Autodesk Fusion 360 part; units mm, degrees
(part 6 of 14)
  line L3010 (-202.4856, -153.9875) -> (-196.9863, -163.5125)
  line L3011 (-196.9863, -163.5125) -> (-185.9878, -163.5125)
  line L3012 (-180.4886, -153.9875) -> (-185.9878, -144.4625)
  line L3013 (-185.9878, -163.5125) -> (-180.4886, -153.9875)
  line L3014 (-166.7404, -133.35) -> (-177.7389, -133.35)
  line L3015 (-177.7389, -133.35) -> (-183.2382, -142.875)
  line L3016 (-183.2382, -142.875) -> (-177.7389, -152.4)
  line L3017 (-177.7389, -152.4) -> (-166.7404, -152.4)
  line L3018 (-161.2411, -142.875) -> (-166.7404, -133.35)
  line L3019 (-166.7404, -152.4) -> (-161.2411, -142.875)
  line L3020 (-147.493, -122.2375) -> (-158.4915, -122.2375)
  line L3021 (-158.4915, -122.2375) -> (-163.9908, -131.7625)
  line L3022 (-163.9908, -131.7625) -> (-158.4915, -141.2875)
  line L3023 (-158.4915, -141.2875) -> (-147.493, -141.2875)
  line L3024 (-141.9937, -131.7625) -> (-147.493, -122.2375)
  line L3025 (-147.493, -141.2875) -> (-141.9937, -131.7625)
  line L3026 (-128.2456, -111.125) -> (-139.2441, -111.125)
  line L3027 (-139.2441, -111.125) -> (-144.7434, -120.65)
  line L3028 (-144.7434, -120.65) -> (-139.2441, -130.175)
  line L3029 (-139.2441, -130.175) -> (-128.2456, -130.175)
  line L3030 (-122.7463, -120.65) -> (-128.2456, -111.125)
  line L3031 (-128.2456, -130.175) -> (-122.7463, -120.65)
  line L3032 (-108.9982, -100.0125) -> (-119.9967, -100.0125)
  line L3033 (-119.9967, -100.0125) -> (-125.4959, -109.5375)
  line L3034 (-125.4959, -109.5375) -> (-119.9967, -119.0625)
  line L3035 (-119.9967, -119.0625) -> (-108.9982, -119.0625)
  line L3036 (-103.4989, -109.5375) -> (-108.9982, -100.0125)
  line L3037 (-108.9982, -119.0625) -> (-103.4989, -109.5375)
  line L3038 (-89.7507, -88.9) -> (-100.7493, -88.9)
  line L3039 (-100.7493, -88.9) -> (-106.2485, -98.425)
  line L3040 (-106.2485, -98.425) -> (-100.7493, -107.95)
  line L3041 (-100.7493, -107.95) -> (-89.7507, -107.95)
  line L3042 (-84.2515, -98.425) -> (-89.7507, -88.9)
  line L3043 (-89.7507, -107.95) -> (-84.2515, -98.425)
  line L3044 (-70.5033, -77.7875) -> (-81.5018, -77.7875)
  line L3045 (-81.5018, -77.7875) -> (-87.0011, -87.3125)
  line L3046 (-87.0011, -87.3125) -> (-81.5018, -96.8375)
  line L3047 (-81.5018, -96.8375) -> (-70.5033, -96.8375)
  line L3048 (-65.0041, -87.3125) -> (-70.5033, -77.7875)
  line L3049 (-70.5033, -96.8375) -> (-65.0041, -87.3125)
  line L3050 (-51.2559, -66.675) -> (-62.2544, -66.675)
  line L3051 (-62.2544, -66.675) -> (-67.7537, -76.2)
  line L3052 (-67.7537, -76.2) -> (-62.2544, -85.725)
  line L3053 (-62.2544, -85.725) -> (-51.2559, -85.725)
  line L3054 (-45.7566, -76.2) -> (-51.2559, -66.675)
  line L3055 (-51.2559, -85.725) -> (-45.7566, -76.2)
  line L3056 (-32.0085, -55.5625) -> (-43.007, -55.5625)
  line L3057 (-43.007, -55.5625) -> (-48.5063, -65.0875)
  line L3058 (-48.5063, -65.0875) -> (-43.007, -74.6125)
  line L3059 (-43.007, -74.6125) -> (-32.0085, -74.6125)
  line L3060 (-26.5092, -65.0875) -> (-32.0085, -55.5625)
  line L3061 (-32.0085, -74.6125) -> (-26.5092, -65.0875)
  line L3062 (-12.7611, -44.45) -> (-23.7596, -44.45)
  line L3063 (-23.7596, -44.45) -> (-29.2589, -53.975)
  line L3064 (-29.2589, -53.975) -> (-23.7596, -63.5)
  line L3065 (-23.7596, -63.5) -> (-12.7611, -63.5)
  line L3066 (-7.2618, -53.975) -> (-12.7611, -44.45)
  line L3067 (-12.7611, -63.5) -> (-7.2618, -53.975)
  line L3068 (6.4863, -33.3375) -> (-4.5122, -33.3375)
  line L3069 (-4.5122, -33.3375) -> (-10.0114, -42.8625)
  line L3070 (-10.0114, -42.8625) -> (-4.5122, -52.3875)
  line L3071 (-4.5122, -52.3875) -> (6.4863, -52.3875)
  line L3072 (11.9856, -42.8625) -> (6.4863, -33.3375)
  line L3073 (6.4863, -52.3875) -> (11.9856, -42.8625)
  line L3074 (25.7337, -22.225) -> (14.7352, -22.225)
  line L3075 (14.7352, -22.225) -> (9.236, -31.75)
  line L3076 (9.236, -31.75) -> (14.7352, -41.275)
  line L3077 (14.7352, -41.275) -> (25.7337, -41.275)
  line L3078 (31.233, -31.75) -> (25.7337, -22.225)
  line L3079 (25.7337, -41.275) -> (31.233, -31.75)
  line L3080 (44.9812, -11.1125) -> (33.9826, -11.1125)
  line L3081 (33.9826, -11.1125) -> (28.4834, -20.6375)
  line L3082 (28.4834, -20.6375) -> (33.9826, -30.1625)
  line L3083 (33.9826, -30.1625) -> (44.9812, -30.1625)
  line L3084 (50.4804, -20.6375) -> (44.9812, -11.1125)
  line L3085 (44.9812, -30.1625) -> (50.4804, -20.6375)
  line L3086 (64.2286, 0) -> (53.2301, 0)
  line L3087 (53.2301, 0) -> (47.7308, -9.525)
  line L3088 (47.7308, -9.525) -> (53.2301, -19.05)
  line L3089 (53.2301, -19.05) -> (64.2286, -19.05)
  line L3090 (69.7278, -9.525) -> (64.2286, 0)
  line L3091 (64.2286, -19.05) -> (69.7278, -9.525)
  line L3092 (83.476, 11.1125) -> (72.4775, 11.1125)
  line L3093 (72.4775, 11.1125) -> (66.9782, 1.5875)
  line L3094 (66.9782, 1.5875) -> (72.4775, -7.9375)
  line L3095 (72.4775, -7.9375) -> (83.476, -7.9375)
  line L3096 (88.9753, 1.5875) -> (83.476, 11.1125)
  line L3097 (83.476, -7.9375) -> (88.9753, 1.5875)
  line L3098 (102.7234, 22.225) -> (91.7249, 22.225)
  line L3099 (91.7249, 22.225) -> (86.2256, 12.7)
  line L3100 (86.2256, 12.7) -> (91.7249, 3.175)
  line L3101 (91.7249, 3.175) -> (102.7234, 3.175)
  line L3102 (108.2227, 12.7) -> (102.7234, 22.225)
  line L3103 (102.7234, 3.175) -> (108.2227, 12.7)
  line L3104 (121.9708, 33.3375) -> (110.9723, 33.3375)
  line L3105 (110.9723, 33.3375) -> (105.473, 23.8125)
  line L3106 (105.473, 23.8125) -> (110.9723, 14.2875)
  line L3107 (110.9723, 14.2875) -> (121.9708, 14.2875)
  line L3108 (127.4701, 23.8125) -> (121.9708, 33.3375)
  line L3109 (121.9708, 14.2875) -> (127.4701, 23.8125)
  line L3110 (141.2182, 44.45) -> (130.2197, 44.45)
  line L3111 (130.2197, 44.45) -> (124.7205, 34.925)
  line L3112 (124.7205, 34.925) -> (130.2197, 25.4)
  line L3113 (130.2197, 25.4) -> (141.2182, 25.4)
  line L3114 (146.7175, 34.925) -> (141.2182, 44.45)
  line L3115 (141.2182, 25.4) -> (146.7175, 34.925)
  line L3116 (160.4657, 55.5625) -> (149.4671, 55.5625)
  line L3117 (149.4671, 55.5625) -> (143.9679, 46.0375)
  line L3118 (143.9679, 46.0375) -> (149.4671, 36.5125)
  line L3119 (149.4671, 36.5125) -> (160.4657, 36.5125)
  line L3120 (165.9649, 46.0375) -> (160.4657, 55.5625)
  line L3121 (160.4657, 36.5125) -> (165.9649, 46.0375)
  line L3122 (179.7131, 66.675) -> (168.7145, 66.675)
  line L3123 (168.7145, 66.675) -> (163.2153, 57.15)
  line L3124 (163.2153, 57.15) -> (168.7145, 47.625)
  line L3125 (168.7145, 47.625) -> (179.7131, 47.625)
  line L3126 (185.2123, 57.15) -> (179.7131, 66.675)
  line L3127 (179.7131, 47.625) -> (185.2123, 57.15)
  line L3128 (198.9605, 77.7875) -> (187.962, 77.7875)
  line L3129 (187.962, 77.7875) -> (182.4627, 68.2625)
  line L3130 (182.4627, 68.2625) -> (187.962, 58.7375)
  line L3131 (187.962, 58.7375) -> (198.9605, 58.7375)
  line L3132 (204.4597, 68.2625) -> (198.9605, 77.7875)
  line L3133 (198.9605, 58.7375) -> (204.4597, 68.2625)
  line L3134 (218.2079, 88.9) -> (207.2094, 88.9)
  line L3135 (207.2094, 88.9) -> (201.7101, 79.375)
  line L3136 (201.7101, 79.375) -> (207.2094, 69.85)
  line L3137 (207.2094, 69.85) -> (218.2079, 69.85)
  line L3138 (223.7072, 79.375) -> (218.2079, 88.9)
  line L3139 (218.2079, 69.85) -> (223.7072, 79.375)
  line L3140 (237.4553, 100.0125) -> (226.4568, 100.0125)
  line L3141 (226.4568, 100.0125) -> (220.9575, 90.4875)
  line L3142 (220.9575, 90.4875) -> (226.4568, 80.9625)
  line L3143 (226.4568, 80.9625) -> (237.4553, 80.9625)
  line L3144 (242.9546, 90.4875) -> (237.4553, 100.0125)
  line L3145 (237.4553, 80.9625) -> (242.9546, 90.4875)
  line L3146 (256.7027, 111.125) -> (245.7042, 111.125)
  line L3147 (245.7042, 111.125) -> (240.2049, 101.6)
  line L3148 (240.2049, 101.6) -> (245.7042, 92.075)
  line L3149 (245.7042, 92.075) -> (256.7027, 92.075)
  line L3150 (262.202, 101.6) -> (256.7027, 111.125)
  line L3151 (256.7027, 92.075) -> (262.202, 101.6)
  line L3152 (275.9501, 122.2375) -> (264.9516, 122.2375)
  line L3153 (264.9516, 122.2375) -> (259.4524, 112.7125)
  line L3154 (259.4524, 112.7125) -> (264.9516, 103.1875)
  line L3155 (264.9516, 103.1875) -> (275.9501, 103.1875)
  line L3156 (281.4494, 112.7125) -> (275.9501, 122.2375)
  line L3157 (275.9501, 103.1875) -> (281.4494, 112.7125)
  line L3158 (295.1976, 133.35) -> (284.199, 133.35)
  line L3159 (284.199, 133.35) -> (278.6998, 123.825)
  line L3160 (278.6998, 123.825) -> (284.199, 114.3)
  line L3161 (284.199, 114.3) -> (295.1976, 114.3)
  line L3162 (300.6968, 123.825) -> (295.1976, 133.35)
  line L3163 (295.1976, 114.3) -> (300.6968, 123.825)
  line L3164 (314.445, 144.4625) -> (303.4464, 144.4625)
  line L3165 (303.4464, 144.4625) -> (297.9472, 134.9375)
  line L3166 (297.9472, 134.9375) -> (303.4464, 125.4125)
  line L3167 (303.4464, 125.4125) -> (314.445, 125.4125)
  line L3168 (319.9442, 134.9375) -> (314.445, 144.4625)
  line L3169 (314.445, 125.4125) -> (319.9442, 134.9375)
  line L3170 (333.6924, 155.575) -> (322.6939, 155.575)
  line L3171 (322.6939, 155.575) -> (317.1946, 146.05)
  line L3172 (317.1946, 146.05) -> (322.6939, 136.525)
  line L3173 (322.6939, 136.525) -> (333.6924, 136.525)
  line L3174 (339.1916, 146.05) -> (333.6924, 155.575)
  line L3175 (333.6924, 136.525) -> (339.1916, 146.05)
  line L3176 (352.9398, 166.6875) -> (341.9413, 166.6875)
  line L3177 (341.9413, 166.6875) -> (336.442, 157.1625)
  line L3178 (336.442, 157.1625) -> (341.9413, 147.6375)
  line L3179 (341.9413, 147.6375) -> (352.9398, 147.6375)
  line L3180 (358.4391, 157.1625) -> (352.9398, 166.6875)
  line L3181 (352.9398, 147.6375) -> (358.4391, 157.1625)
  line L3182 (372.1872, 177.8) -> (361.1887, 177.8)
  line L3183 (361.1887, 177.8) -> (355.6894, 168.275)
  line L3184 (355.6894, 168.275) -> (361.1887, 158.75)
  line L3185 (361.1887, 158.75) -> (372.1872, 158.75)
  line L3186 (377.6865, 168.275) -> (372.1872, 177.8)
  line L3187 (372.1872, 158.75) -> (377.6865, 168.275)
  line L3188 (391.4346, 188.9125) -> (380.4361, 188.9125)
  line L3189 (380.4361, 188.9125) -> (374.9368, 179.3875)
  line L3190 (374.9368, 179.3875) -> (380.4361, 169.8625)
  line L3191 (380.4361, 169.8625) -> (391.4346, 169.8625)
  line L3192 (396.9339, 179.3875) -> (391.4346, 188.9125)
  line L3193 (391.4346, 169.8625) -> (396.9339, 179.3875)
  line L3194 (410.682, 200.025) -> (399.6835, 200.025)
  line L3195 (399.6835, 200.025) -> (394.1843, 190.5)
  line L3196 (394.1843, 190.5) -> (399.6835, 180.975)
  line L3197 (399.6835, 180.975) -> (410.682, 180.975)
  line L3198 (416.1813, 190.5) -> (410.682, 200.025)
  line L3199 (410.682, 180.975) -> (416.1813, 190.5)
  line L3200 (429.9295, 211.1375) -> (418.9309, 211.1375)
  line L3201 (418.9309, 211.1375) -> (413.4317, 201.6125)
  line L3202 (413.4317, 201.6125) -> (418.9309, 192.0875)
  line L3203 (418.9309, 192.0875) -> (429.9295, 192.0875)
  line L3204 (435.4287, 201.6125) -> (429.9295, 211.1375)
  line L3205 (429.9295, 192.0875) -> (435.4287, 201.6125)
  line L3206 (449.1769, 222.25) -> (438.1783, 222.25)
  line L3207 (438.1783, 222.25) -> (432.6791, 212.725)
  line L3208 (432.6791, 212.725) -> (438.1783, 203.2)
  line L3209 (438.1783, 203.2) -> (449.1769, 203.2)
  line L3210 (454.6761, 212.725) -> (449.1769, 222.25)
  line L3211 (449.1769, 203.2) -> (454.6761, 212.725)
  line L3212 (468.4243, 233.3625) -> (457.4258, 233.3625)
  line L3213 (457.4258, 233.3625) -> (451.9265, 223.8375)
  line L3214 (451.9265, 223.8375) -> (457.4258, 214.3125)
  line L3215 (457.4258, 214.3125) -> (468.4243, 214.3125)
  line L3216 (473.9235, 223.8375) -> (468.4243, 233.3625)
  line L3217 (468.4243, 214.3125) -> (473.9235, 223.8375)
  line L3218 (487.6717, 244.475) -> (476.6732, 244.475)
  line L3219 (476.6732, 244.475) -> (471.1739, 234.95)
  line L3220 (471.1739, 234.95) -> (476.6732, 225.425)
  line L3221 (476.6732, 225.425) -> (487.6717, 225.425)
  line L3222 (493.171, 234.95) -> (487.6717, 244.475)
  line L3223 (487.6717, 225.425) -> (493.171, 234.95)
  line L3224 (506.9191, 255.5875) -> (495.9206, 255.5875)
  line L3225 (495.9206, 255.5875) -> (490.4213, 246.0625)
  line L3226 (490.4213, 246.0625) -> (495.9206, 236.5375)
  line L3227 (495.9206, 236.5375) -> (506.9191, 236.5375)
  line L3228 (512.4184, 246.0625) -> (506.9191, 255.5875)
  line L3229 (506.9191, 236.5375) -> (512.4184, 246.0625)
  line L3230 (526.1665, 266.7) -> (515.168, 266.7)
  line L3231 (515.168, 266.7) -> (509.6687, 257.175)
  line L3232 (509.6687, 257.175) -> (515.168, 247.65)
  line L3233 (515.168, 247.65) -> (526.1665, 247.65)
  line L3234 (531.6658, 257.175) -> (526.1665, 266.7)
  line L3235 (526.1665, 247.65) -> (531.6658, 257.175)
  line L3236 (545.4139, 277.8125) -> (534.4154, 277.8125)
  line L3237 (534.4154, 277.8125) -> (528.9162, 268.2875)
  line L3238 (528.9162, 268.2875) -> (534.4154, 258.7625)
  line L3239 (534.4154, 258.7625) -> (545.4139, 258.7625)
  line L3240 (550.9132, 268.2875) -> (545.4139, 277.8125)
  line L3241 (545.4139, 258.7625) -> (550.9132, 268.2875)
  line L3242 (564.6614, 288.925) -> (553.6628, 288.925)
  line L3243 (553.6628, 288.925) -> (548.1636, 279.4)
  line L3244 (548.1636, 279.4) -> (553.6628, 269.875)
  line L3245 (553.6628, 269.875) -> (564.6614, 269.875)
  line L3246 (570.1606, 279.4) -> (564.6614, 288.925)
  line L3247 (564.6614, 269.875) -> (570.1606, 279.4)
  line L3248 (583.9088, 300.0375) -> (572.9102, 300.0375)
  line L3249 (572.9102, 300.0375) -> (567.411, 290.5125)
  line L3250 (567.411, 290.5125) -> (572.9102, 280.9875)
  line L3251 (572.9102, 280.9875) -> (583.9088, 280.9875)
  line L3252 (589.408, 290.5125) -> (583.9088, 300.0375)
  line L3253 (583.9088, 280.9875) -> (589.408, 290.5125)
  line L3254 (603.1562, 311.15) -> (592.1577, 311.15)
  line L3255 (592.1577, 311.15) -> (586.6584, 301.625)
  line L3256 (586.6584, 301.625) -> (592.1577, 292.1)
  line L3257 (592.1577, 292.1) -> (603.1562, 292.1)
  line L3258 (608.6554, 301.625) -> (603.1562, 311.15)
  line L3259 (603.1562, 292.1) -> (608.6554, 301.625)
  line L3260 (-551.6887, -333.375) -> (-562.6872, -333.375)
  line L3261 (-562.6872, -333.375) -> (-568.1865, -342.9)
  line L3262 (-568.1865, -342.9) -> (-562.6872, -352.425)
  line L3263 (-562.6872, -352.425) -> (-551.6887, -352.425)
  line L3264 (-546.1894, -342.9) -> (-551.6887, -333.375)
  line L3265 (-551.6887, -352.425) -> (-546.1894, -342.9)
  line L3266 (-532.4413, -322.2625) -> (-543.4398, -322.2625)
  line L3267 (-543.4398, -322.2625) -> (-548.9391, -331.7875)
  line L3268 (-548.9391, -331.7875) -> (-543.4398, -341.3125)
  line L3269 (-543.4398, -341.3125) -> (-532.4413, -341.3125)
  line L3270 (-526.942, -331.7875) -> (-532.4413, -322.2625)
  line L3271 (-532.4413, -341.3125) -> (-526.942, -331.7875)
  line L3272 (-513.1939, -311.15) -> (-524.1924, -311.15)
  line L3273 (-524.1924, -311.15) -> (-529.6916, -320.675)
  line L3274 (-529.6916, -320.675) -> (-524.1924, -330.2)
  line L3275 (-524.1924, -330.2) -> (-513.1939, -330.2)
  line L3276 (-507.6946, -320.675) -> (-513.1939, -311.15)
  line L3277 (-513.1939, -330.2) -> (-507.6946, -320.675)
  line L3278 (-493.9464, -300.0375) -> (-504.945, -300.0375)
  line L3279 (-504.945, -300.0375) -> (-510.4442, -309.5625)
  line L3280 (-510.4442, -309.5625) -> (-504.945, -319.0875)
  line L3281 (-504.945, -319.0875) -> (-493.9464, -319.0875)
  line L3282 (-488.4472, -309.5625) -> (-493.9464, -300.0375)
  line L3283 (-493.9464, -319.0875) -> (-488.4472, -309.5625)
  line L3284 (-474.699, -288.925) -> (-485.6976, -288.925)
  line L3285 (-485.6976, -288.925) -> (-491.1968, -298.45)
  line L3286 (-491.1968, -298.45) -> (-485.6976, -307.975)
  line L3287 (-485.6976, -307.975) -> (-474.699, -307.975)
  line L3288 (-469.1998, -298.45) -> (-474.699, -288.925)
  line L3289 (-474.699, -307.975) -> (-469.1998, -298.45)
  line L3290 (-455.4516, -277.8125) -> (-466.4501, -277.8125)
  line L3291 (-466.4501, -277.8125) -> (-471.9494, -287.3375)
  line L3292 (-471.9494, -287.3375) -> (-466.4501, -296.8625)
  line L3293 (-466.4501, -296.8625) -> (-455.4516, -296.8625)
  line L3294 (-449.9524, -287.3375) -> (-455.4516, -277.8125)
  line L3295 (-455.4516, -296.8625) -> (-449.9524, -287.3375)
  line L3296 (-436.2042, -266.7) -> (-447.2027, -266.7)
  line L3297 (-447.2027, -266.7) -> (-452.702, -276.225)
  line L3298 (-452.702, -276.225) -> (-447.2027, -285.75)
  line L3299 (-447.2027, -285.75) -> (-436.2042, -285.75)
  line L3300 (-430.7049, -276.225) -> (-436.2042, -266.7)
  line L3301 (-436.2042, -285.75) -> (-430.7049, -276.225)
  line L3302 (-416.9568, -255.5875) -> (-427.9553, -255.5875)
  line L3303 (-427.9553, -255.5875) -> (-433.4546, -265.1125)
  line L3304 (-433.4546, -265.1125) -> (-427.9553, -274.6375)
  line L3305 (-427.9553, -274.6375) -> (-416.9568, -274.6375)
  line L3306 (-411.4575, -265.1125) -> (-416.9568, -255.5875)
  line L3307 (-416.9568, -274.6375) -> (-411.4575, -265.1125)
  line L3308 (-397.7094, -244.475) -> (-408.7079, -244.475)
  line L3309 (-408.7079, -244.475) -> (-414.2072, -254)
  line L3310 (-414.2072, -254) -> (-408.7079, -263.525)
  line L3311 (-408.7079, -263.525) -> (-397.7094, -263.525)
  line L3312 (-392.2101, -254) -> (-397.7094, -244.475)
  line L3313 (-397.7094, -263.525) -> (-392.2101, -254)
  line L3314 (-378.462, -233.3625) -> (-389.4605, -233.3625)
  line L3315 (-389.4605, -233.3625) -> (-394.9597, -242.8875)
  line L3316 (-394.9597, -242.8875) -> (-389.4605, -252.4125)
  line L3317 (-389.4605, -252.4125) -> (-378.462, -252.4125)
  line L3318 (-372.9627, -242.8875) -> (-378.462, -233.3625)
  line L3319 (-378.462, -252.4125) -> (-372.9627, -242.8875)
  line L3320 (-359.2145, -222.25) -> (-370.2131, -222.25)
  line L3321 (-370.2131, -222.25) -> (-375.7123, -231.775)
  line L3322 (-375.7123, -231.775) -> (-370.2131, -241.3)
  line L3323 (-370.2131, -241.3) -> (-359.2145, -241.3)
  line L3324 (-353.7153, -231.775) -> (-359.2145, -222.25)
  line L3325 (-359.2145, -241.3) -> (-353.7153, -231.775)
  line L3326 (-339.9671, -211.1375) -> (-350.9657, -211.1375)
  line L3327 (-350.9657, -211.1375) -> (-356.4649, -220.6625)
  line L3328 (-356.4649, -220.6625) -> (-350.9657, -230.1875)
  line L3329 (-350.9657, -230.1875) -> (-339.9671, -230.1875)
  line L3330 (-334.4679, -220.6625) -> (-339.9671, -211.1375)
  line L3331 (-339.9671, -230.1875) -> (-334.4679, -220.6625)
  line L3332 (-320.7197, -200.025) -> (-331.7182, -200.025)
  line L3333 (-331.7182, -200.025) -> (-337.2175, -209.55)
  line L3334 (-337.2175, -209.55) -> (-331.7182, -219.075)
  line L3335 (-331.7182, -219.075) -> (-320.7197, -219.075)
  line L3336 (-315.2205, -209.55) -> (-320.7197, -200.025)
  line L3337 (-320.7197, -219.075) -> (-315.2205, -209.55)
  line L3338 (-301.4723, -188.9125) -> (-312.4708, -188.9125)
  line L3339 (-312.4708, -188.9125) -> (-317.9701, -198.4375)
  line L3340 (-317.9701, -198.4375) -> (-312.4708, -207.9625)
  line L3341 (-312.4708, -207.9625) -> (-301.4723, -207.9625)
  line L3342 (-295.973, -198.4375) -> (-301.4723, -188.9125)
  line L3343 (-301.4723, -207.9625) -> (-295.973, -198.4375)
  line L3344 (-282.2249, -177.8) -> (-293.2234, -177.8)
  line L3345 (-293.2234, -177.8) -> (-298.7227, -187.325)
  line L3346 (-298.7227, -187.325) -> (-293.2234, -196.85)
  line L3347 (-293.2234, -196.85) -> (-282.2249, -196.85)
  line L3348 (-276.7256, -187.325) -> (-282.2249, -177.8)
  line L3349 (-282.2249, -196.85) -> (-276.7256, -187.325)
  line L3350 (-262.9775, -166.6875) -> (-273.976, -166.6875)
  line L3351 (-273.976, -166.6875) -> (-279.4753, -176.2125)
  line L3352 (-279.4753, -176.2125) -> (-273.976, -185.7375)
  line L3353 (-273.976, -185.7375) -> (-262.9775, -185.7375)
  line L3354 (-257.4782, -176.2125) -> (-262.9775, -166.6875)
  line L3355 (-262.9775, -185.7375) -> (-257.4782, -176.2125)
  line L3356 (-243.7301, -155.575) -> (-254.7286, -155.575)
  line L3357 (-254.7286, -155.575) -> (-260.2278, -165.1)
  line L3358 (-260.2278, -165.1) -> (-254.7286, -174.625)
  line L3359 (-254.7286, -174.625) -> (-243.7301, -174.625)
  line L3360 (-238.2308, -165.1) -> (-243.7301, -155.575)
  line L3361 (-243.7301, -174.625) -> (-238.2308, -165.1)
  line L3362 (-224.4826, -144.4625) -> (-235.4812, -144.4625)
  line L3363 (-235.4812, -144.4625) -> (-240.9804, -153.9875)
  line L3364 (-240.9804, -153.9875) -> (-235.4812, -163.5125)
  line L3365 (-235.4812, -163.5125) -> (-224.4826, -163.5125)
  line L3366 (-218.9834, -153.9875) -> (-224.4826, -144.4625)
  line L3367 (-224.4826, -163.5125) -> (-218.9834, -153.9875)
  line L3368 (-205.2352, -133.35) -> (-216.2337, -133.35)
  line L3369 (-216.2337, -133.35) -> (-221.733, -142.875)
  line L3370 (-221.733, -142.875) -> (-216.2337, -152.4)
  line L3371 (-216.2337, -152.4) -> (-205.2352, -152.4)
  line L3372 (-199.736, -142.875) -> (-205.2352, -133.35)
  line L3373 (-205.2352, -152.4) -> (-199.736, -142.875)
  line L3374 (-185.9878, -122.2375) -> (-196.9863, -122.2375)
  line L3375 (-196.9863, -122.2375) -> (-202.4856, -131.7625)
  line L3376 (-202.4856, -131.7625) -> (-196.9863, -141.2875)
  line L3377 (-196.9863, -141.2875) -> (-185.9878, -141.2875)
  line L3378 (-180.4886, -131.7625) -> (-185.9878, -122.2375)
  line L3379 (-185.9878, -141.2875) -> (-180.4886, -131.7625)
  line L3380 (-166.7404, -111.125) -> (-177.7389, -111.125)
  line L3381 (-177.7389, -111.125) -> (-183.2382, -120.65)
  line L3382 (-183.2382, -120.65) -> (-177.7389, -130.175)
  line L3383 (-177.7389, -130.175) -> (-166.7404, -130.175)
  line L3384 (-161.2411, -120.65) -> (-166.7404, -111.125)
  line L3385 (-166.7404, -130.175) -> (-161.2411, -120.65)
  line L3386 (-147.493, -100.0125) -> (-158.4915, -100.0125)
  line L3387 (-158.4915, -100.0125) -> (-163.9908, -109.5375)
  line L3388 (-163.9908, -109.5375) -> (-158.4915, -119.0625)
  line L3389 (-158.4915, -119.0625) -> (-147.493, -119.0625)
  line L3390 (-141.9937, -109.5375) -> (-147.493, -100.0125)
  line L3391 (-147.493, -119.0625) -> (-141.9937, -109.5375)
  line L3392 (-128.2456, -88.9) -> (-139.2441, -88.9)
  line L3393 (-139.2441, -88.9) -> (-144.7434, -98.425)
  line L3394 (-144.7434, -98.425) -> (-139.2441, -107.95)
  line L3395 (-139.2441, -107.95) -> (-128.2456, -107.95)
  line L3396 (-122.7463, -98.425) -> (-128.2456, -88.9)
  line L3397 (-128.2456, -107.95) -> (-122.7463, -98.425)
  line L3398 (-108.9982, -77.7875) -> (-119.9967, -77.7875)
  line L3399 (-119.9967, -77.7875) -> (-125.4959, -87.3125)
  line L3400 (-125.4959, -87.3125) -> (-119.9967, -96.8375)
  line L3401 (-119.9967, -96.8375) -> (-108.9982, -96.8375)
  line L3402 (-103.4989, -87.3125) -> (-108.9982, -77.7875)
  line L3403 (-108.9982, -96.8375) -> (-103.4989, -87.3125)
  line L3404 (-89.7507, -66.675) -> (-100.7493, -66.675)
  line L3405 (-100.7493, -66.675) -> (-106.2485, -76.2)
  line L3406 (-106.2485, -76.2) -> (-100.7493, -85.725)
  line L3407 (-100.7493, -85.725) -> (-89.7507, -85.725)
  line L3408 (-84.2515, -76.2) -> (-89.7507, -66.675)
  line L3409 (-89.7507, -85.725) -> (-84.2515, -76.2)
  line L3410 (-70.5033, -55.5625) -> (-81.5018, -55.5625)
  line L3411 (-81.5018, -55.5625) -> (-87.0011, -65.0875)
  line L3412 (-87.0011, -65.0875) -> (-81.5018, -74.6125)
  line L3413 (-81.5018, -74.6125) -> (-70.5033, -74.6125)
  line L3414 (-65.0041, -65.0875) -> (-70.5033, -55.5625)
  line L3415 (-70.5033, -74.6125) -> (-65.0041, -65.0875)
  line L3416 (-51.2559, -44.45) -> (-62.2544, -44.45)
  line L3417 (-62.2544, -44.45) -> (-67.7537, -53.975)
  line L3418 (-67.7537, -53.975) -> (-62.2544, -63.5)
  line L3419 (-62.2544, -63.5) -> (-51.2559, -63.5)
  line L3420 (-45.7566, -53.975) -> (-51.2559, -44.45)
  line L3421 (-51.2559, -63.5) -> (-45.7566, -53.975)
  line L3422 (-32.0085, -33.3375) -> (-43.007, -33.3375)
  line L3423 (-43.007, -33.3375) -> (-48.5063, -42.8625)
  line L3424 (-48.5063, -42.8625) -> (-43.007, -52.3875)
  line L3425 (-43.007, -52.3875) -> (-32.0085, -52.3875)
  line L3426 (-26.5092, -42.8625) -> (-32.0085, -33.3375)
  line L3427 (-32.0085, -52.3875) -> (-26.5092, -42.8625)
  line L3428 (-12.7611, -22.225) -> (-23.7596, -22.225)
  line L3429 (-23.7596, -22.225) -> (-29.2589, -31.75)
  line L3430 (-29.2589, -31.75) -> (-23.7596, -41.275)
  line L3431 (-23.7596, -41.275) -> (-12.7611, -41.275)
  line L3432 (-7.2618, -31.75) -> (-12.7611, -22.225)
  line L3433 (-12.7611, -41.275) -> (-7.2618, -31.75)
  line L3434 (6.4863, -11.1125) -> (-4.5122, -11.1125)
  line L3435 (-4.5122, -11.1125) -> (-10.0114, -20.6375)
  line L3436 (-10.0114, -20.6375) -> (-4.5122, -30.1625)
  line L3437 (-4.5122, -30.1625) -> (6.4863, -30.1625)
  line L3438 (11.9856, -20.6375) -> (6.4863, -11.1125)
  line L3439 (6.4863, -30.1625) -> (11.9856, -20.6375)
  line L3440 (25.7337, 0) -> (14.7352, 0)
  line L3441 (14.7352, 0) -> (9.236, -9.525)
  line L3442 (9.236, -9.525) -> (14.7352, -19.05)
  line L3443 (14.7352, -19.05) -> (25.7337, -19.05)
  line L3444 (31.233, -9.525) -> (25.7337, 0)
  line L3445 (25.7337, -19.05) -> (31.233, -9.525)
  line L3446 (44.9812, 11.1125) -> (33.9826, 11.1125)
  line L3447 (33.9826, 11.1125) -> (28.4834, 1.5875)
  line L3448 (28.4834, 1.5875) -> (33.9826, -7.9375)
  line L3449 (33.9826, -7.9375) -> (44.9812, -7.9375)
  line L3450 (50.4804, 1.5875) -> (44.9812, 11.1125)
  line L3451 (44.9812, -7.9375) -> (50.4804, 1.5875)
  line L3452 (64.2286, 22.225) -> (53.2301, 22.225)
  line L3453 (53.2301, 22.225) -> (47.7308, 12.7)
  line L3454 (47.7308, 12.7) -> (53.2301, 3.175)
  line L3455 (53.2301, 3.175) -> (64.2286, 3.175)
  line L3456 (69.7278, 12.7) -> (64.2286, 22.225)
  line L3457 (64.2286, 3.175) -> (69.7278, 12.7)
  line L3458 (83.476, 33.3375) -> (72.4775, 33.3375)
  line L3459 (72.4775, 33.3375) -> (66.9782, 23.8125)
  line L3460 (66.9782, 23.8125) -> (72.4775, 14.2875)
  line L3461 (72.4775, 14.2875) -> (83.476, 14.2875)
  line L3462 (88.9753, 23.8125) -> (83.476, 33.3375)
  line L3463 (83.476, 14.2875) -> (88.9753, 23.8125)
  line L3464 (102.7234, 44.45) -> (91.7249, 44.45)
  line L3465 (91.7249, 44.45) -> (86.2256, 34.925)
  line L3466 (86.2256, 34.925) -> (91.7249, 25.4)
  line L3467 (91.7249, 25.4) -> (102.7234, 25.4)
  line L3468 (108.2227, 34.925) -> (102.7234, 44.45)
  line L3469 (102.7234, 25.4) -> (108.2227, 34.925)
  line L3470 (121.9708, 55.5625) -> (110.9723, 55.5625)
  line L3471 (110.9723, 55.5625) -> (105.473, 46.0375)
  line L3472 (105.473, 46.0375) -> (110.9723, 36.5125)
  line L3473 (110.9723, 36.5125) -> (121.9708, 36.5125)
  line L3474 (127.4701, 46.0375) -> (121.9708, 55.5625)
  line L3475 (121.9708, 36.5125) -> (127.4701, 46.0375)
  line L3476 (141.2182, 66.675) -> (130.2197, 66.675)
  line L3477 (130.2197, 66.675) -> (124.7205, 57.15)
  line L3478 (124.7205, 57.15) -> (130.2197, 47.625)
  line L3479 (130.2197, 47.625) -> (141.2182, 47.625)
  line L3480 (146.7175, 57.15) -> (141.2182, 66.675)
  line L3481 (141.2182, 47.625) -> (146.7175, 57.15)
  line L3482 (160.4657, 77.7875) -> (149.4671, 77.7875)
  line L3483 (149.4671, 77.7875) -> (143.9679, 68.2625)
  line L3484 (143.9679, 68.2625) -> (149.4671, 58.7375)
  line L3485 (149.4671, 58.7375) -> (160.4657, 58.7375)
  line L3486 (165.9649, 68.2625) -> (160.4657, 77.7875)
  line L3487 (160.4657, 58.7375) -> (165.9649, 68.2625)
  line L3488 (179.7131, 88.9) -> (168.7145, 88.9)
  line L3489 (168.7145, 88.9) -> (163.2153, 79.375)
  line L3490 (163.2153, 79.375) -> (168.7145, 69.85)
  line L3491 (168.7145, 69.85) -> (179.7131, 69.85)
  line L3492 (185.2123, 79.375) -> (179.7131, 88.9)
  line L3493 (179.7131, 69.85) -> (185.2123, 79.375)
  line L3494 (198.9605, 100.0125) -> (187.962, 100.0125)
  line L3495 (187.962, 100.0125) -> (182.4627, 90.4875)
  line L3496 (182.4627, 90.4875) -> (187.962, 80.9625)
  line L3497 (187.962, 80.9625) -> (198.9605, 80.9625)
  line L3498 (204.4597, 90.4875) -> (198.9605, 100.0125)
  line L3499 (198.9605, 80.9625) -> (204.4597, 90.4875)
  line L3500 (218.2079, 111.125) -> (207.2094, 111.125)
  line L3501 (207.2094, 111.125) -> (201.7101, 101.6)
  line L3502 (201.7101, 101.6) -> (207.2094, 92.075)
  line L3503 (207.2094, 92.075) -> (218.2079, 92.075)
  line L3504 (223.7072, 101.6) -> (218.2079, 111.125)
  line L3505 (218.2079, 92.075) -> (223.7072, 101.6)
  line L3506 (237.4553, 122.2375) -> (226.4568, 122.2375)
  line L3507 (226.4568, 122.2375) -> (220.9575, 112.7125)
  line L3508 (220.9575, 112.7125) -> (226.4568, 103.1875)
  line L3509 (226.4568, 103.1875) -> (237.4553, 103.1875)
  line L3510 (242.9546, 112.7125) -> (237.4553, 122.2375)
  line L3511 (237.4553, 103.1875) -> (242.9546, 112.7125)
  line L3512 (256.7027, 133.35) -> (245.7042, 133.35)
  line L3513 (245.7042, 133.35) -> (240.2049, 123.825)
  line L3514 (240.2049, 123.825) -> (245.7042, 114.3)
  line L3515 (245.7042, 114.3) -> (256.7027, 114.3)
  line L3516 (262.202, 123.825) -> (256.7027, 133.35)
  line L3517 (256.7027, 114.3) -> (262.202, 123.825)
  line L3518 (275.9501, 144.4625) -> (264.9516, 144.4625)
  line L3519 (264.9516, 144.4625) -> (259.4524, 134.9375)
  line L3520 (259.4524, 134.9375) -> (264.9516, 125.4125)
  line L3521 (264.9516, 125.4125) -> (275.9501, 125.4125)
  line L3522 (281.4494, 134.9375) -> (275.9501, 144.4625)
  line L3523 (275.9501, 125.4125) -> (281.4494, 134.9375)
  line L3524 (295.1976, 155.575) -> (284.199, 155.575)
  line L3525 (284.199, 155.575) -> (278.6998, 146.05)
  line L3526 (278.6998, 146.05) -> (284.199, 136.525)
  line L3527 (284.199, 136.525) -> (295.1976, 136.525)
  line L3528 (300.6968, 146.05) -> (295.1976, 155.575)
  line L3529 (295.1976, 136.525) -> (300.6968, 146.05)
  line L3530 (314.445, 166.6875) -> (303.4464, 166.6875)
  line L3531 (303.4464, 166.6875) -> (297.9472, 157.1625)
  line L3532 (297.9472, 157.1625) -> (303.4464, 147.6375)
  line L3533 (303.4464, 147.6375) -> (314.445, 147.6375)
  line L3534 (319.9442, 157.1625) -> (314.445, 166.6875)
  line L3535 (314.445, 147.6375) -> (319.9442, 157.1625)
  line L3536 (333.6924, 177.8) -> (322.6939, 177.8)
  line L3537 (322.6939, 177.8) -> (317.1946, 168.275)
  line L3538 (317.1946, 168.275) -> (322.6939, 158.75)
  line L3539 (322.6939, 158.75) -> (333.6924, 158.75)
  line L3540 (339.1916, 168.275) -> (333.6924, 177.8)
  line L3541 (333.6924, 158.75) -> (339.1916, 168.275)
  line L3542 (352.9398, 188.9125) -> (341.9413, 188.9125)
  line L3543 (341.9413, 188.9125) -> (336.442, 179.3875)
  line L3544 (336.442, 179.3875) -> (341.9413, 169.8625)
  line L3545 (341.9413, 169.8625) -> (352.9398, 169.8625)
  line L3546 (358.4391, 179.3875) -> (352.9398, 188.9125)
  line L3547 (352.9398, 169.8625) -> (358.4391, 179.3875)
  line L3548 (372.1872, 200.025) -> (361.1887, 200.025)
  line L3549 (361.1887, 200.025) -> (355.6894, 190.5)
  line L3550 (355.6894, 190.5) -> (361.1887, 180.975)
  line L3551 (361.1887, 180.975) -> (372.1872, 180.975)
  line L3552 (377.6865, 190.5) -> (372.1872, 200.025)
  line L3553 (372.1872, 180.975) -> (377.6865, 190.5)
  line L3554 (391.4346, 211.1375) -> (380.4361, 211.1375)
  line L3555 (380.4361, 211.1375) -> (374.9368, 201.6125)
  line L3556 (374.9368, 201.6125) -> (380.4361, 192.0875)
  line L3557 (380.4361, 192.0875) -> (391.4346, 192.0875)
  line L3558 (396.9339, 201.6125) -> (391.4346, 211.1375)
  line L3559 (391.4346, 192.0875) -> (396.9339, 201.6125)
  line L3560 (410.682, 222.25) -> (399.6835, 222.25)
  line L3561 (399.6835, 222.25) -> (394.1843, 212.725)
  line L3562 (394.1843, 212.725) -> (399.6835, 203.2)
  line L3563 (399.6835, 203.2) -> (410.682, 203.2)
  line L3564 (416.1813, 212.725) -> (410.682, 222.25)
  line L3565 (410.682, 203.2) -> (416.1813, 212.725)
  line L3566 (429.9295, 233.3625) -> (418.9309, 233.3625)
  line L3567 (418.9309, 233.3625) -> (413.4317, 223.8375)
  line L3568 (413.4317, 223.8375) -> (418.9309, 214.3125)
  line L3569 (418.9309, 214.3125) -> (429.9295, 214.3125)
  line L3570 (435.4287, 223.8375) -> (429.9295, 233.3625)
  line L3571 (429.9295, 214.3125) -> (435.4287, 223.8375)
  line L3572 (449.1769, 244.475) -> (438.1783, 244.475)
  line L3573 (438.1783, 244.475) -> (432.6791, 234.95)
  line L3574 (432.6791, 234.95) -> (438.1783, 225.425)
  line L3575 (438.1783, 225.425) -> (449.1769, 225.425)
  line L3576 (454.6761, 234.95) -> (449.1769, 244.475)
  line L3577 (449.1769, 225.425) -> (454.6761, 234.95)
  line L3578 (468.4243, 255.5875) -> (457.4258, 255.5875)
  line L3579 (457.4258, 255.5875) -> (451.9265, 246.0625)
  line L3580 (451.9265, 246.0625) -> (457.4258, 236.5375)
  line L3581 (457.4258, 236.5375) -> (468.4243, 236.5375)
  line L3582 (473.9235, 246.0625) -> (468.4243, 255.5875)
  line L3583 (468.4243, 236.5375) -> (473.9235, 246.0625)
  line L3584 (487.6717, 266.7) -> (476.6732, 266.7)
  line L3585 (476.6732, 266.7) -> (471.1739, 257.175)
  line L3586 (471.1739, 257.175) -> (476.6732, 247.65)
  line L3587 (476.6732, 247.65) -> (487.6717, 247.65)
  line L3588 (493.171, 257.175) -> (487.6717, 266.7)
  line L3589 (487.6717, 247.65) -> (493.171, 257.175)
  line L3590 (506.9191, 277.8125) -> (495.9206, 277.8125)
  line L3591 (495.9206, 277.8125) -> (490.4213, 268.2875)
  line L3592 (490.4213, 268.2875) -> (495.9206, 258.7625)
  line L3593 (495.9206, 258.7625) -> (506.9191, 258.7625)
  line L3594 (512.4184, 268.2875) -> (506.9191, 277.8125)
  line L3595 (506.9191, 258.7625) -> (512.4184, 268.2875)
  line L3596 (526.1665, 288.925) -> (515.168, 288.925)
  line L3597 (515.168, 288.925) -> (509.6687, 279.4)
  line L3598 (509.6687, 279.4) -> (515.168, 269.875)
  line L3599 (515.168, 269.875) -> (526.1665, 269.875)
  line L3600 (531.6658, 279.4) -> (526.1665, 288.925)
  line L3601 (526.1665, 269.875) -> (531.6658, 279.4)
  line L3602 (545.4139, 300.0375) -> (534.4154, 300.0375)
  line L3603 (534.4154, 300.0375) -> (528.9162, 290.5125)
  line L3604 (528.9162, 290.5125) -> (534.4154, 280.9875)
  line L3605 (534.4154, 280.9875) -> (545.4139, 280.9875)
  line L3606 (550.9132, 290.5125) -> (545.4139, 300.0375)
  line L3607 (545.4139, 280.9875) -> (550.9132, 290.5125)
  line L3608 (564.6614, 311.15) -> (553.6628, 311.15)
  line L3609 (553.6628, 311.15) -> (548.1636, 301.625)
  line L3610 (548.1636, 301.625) -> (553.6628, 292.1)
  line L3611 (553.6628, 292.1) -> (564.6614, 292.1)
  line L3612 (570.1606, 301.625) -> (564.6614, 311.15)
  line L3613 (564.6614, 292.1) -> (570.1606, 301.625)
  line L3614 (583.9088, 322.2625) -> (572.9102, 322.2625)
  line L3615 (572.9102, 322.2625) -> (567.411, 312.7375)
  line L3616 (567.411, 312.7375) -> (572.9102, 303.2125)
  line L3617 (572.9102, 303.2125) -> (583.9088, 303.2125)
  line L3618 (589.408, 312.7375) -> (583.9088, 322.2625)
  line L3619 (583.9088, 303.2125) -> (589.408, 312.7375)
  line L3620 (-570.9361, -322.2625) -> (-581.9346, -322.2625)
  line L3621 (-581.9346, -322.2625) -> (-587.4339, -331.7875)
  line L3622 (-587.4339, -331.7875) -> (-581.9346, -341.3125)
  line L3623 (-581.9346, -341.3125) -> (-570.9361, -341.3125)
  line L3624 (-565.4368, -331.7875) -> (-570.9361, -322.2625)
  line L3625 (-570.9361, -341.3125) -> (-565.4368, -331.7875)
  line L3626 (-551.6887, -311.15) -> (-562.6872, -311.15)
  line L3627 (-562.6872, -311.15) -> (-568.1865, -320.675)
  line L3628 (-568.1865, -320.675) -> (-562.6872, -330.2)
  line L3629 (-562.6872, -330.2) -> (-551.6887, -330.2)
  line L3630 (-546.1894, -320.675) -> (-551.6887, -311.15)
  line L3631 (-551.6887, -330.2) -> (-546.1894, -320.675)
  line L3632 (-532.4413, -300.0375) -> (-543.4398, -300.0375)
  line L3633 (-543.4398, -300.0375) -> (-548.9391, -309.5625)
  line L3634 (-548.9391, -309.5625) -> (-543.4398, -319.0875)
  line L3635 (-543.4398, -319.0875) -> (-532.4413, -319.0875)
  line L3636 (-526.942, -309.5625) -> (-532.4413, -300.0375)
  line L3637 (-532.4413, -319.0875) -> (-526.942, -309.5625)
  line L3638 (-513.1939, -288.925) -> (-524.1924, -288.925)
  line L3639 (-524.1924, -288.925) -> (-529.6916, -298.45)
  line L3640 (-529.6916, -298.45) -> (-524.1924, -307.975)
  line L3641 (-524.1924, -307.975) -> (-513.1939, -307.975)
  line L3642 (-507.6946, -298.45) -> (-513.1939, -288.925)
  line L3643 (-513.1939, -307.975) -> (-507.6946, -298.45)
  line L3644 (-493.9464, -277.8125) -> (-504.945, -277.8125)
  line L3645 (-504.945, -277.8125) -> (-510.4442, -287.3375)
  line L3646 (-510.4442, -287.3375) -> (-504.945, -296.8625)
  line L3647 (-504.945, -296.8625) -> (-493.9464, -296.8625)
  line L3648 (-488.4472, -287.3375) -> (-493.9464, -277.8125)
  line L3649 (-493.9464, -296.8625) -> (-488.4472, -287.3375)
  line L3650 (-474.699, -266.7) -> (-485.6976, -266.7)
  line L3651 (-485.6976, -266.7) -> (-491.1968, -276.225)
  line L3652 (-491.1968, -276.225) -> (-485.6976, -285.75)
  line L3653 (-485.6976, -285.75) -> (-474.699, -285.75)
  line L3654 (-469.1998, -276.225) -> (-474.699, -266.7)
  line L3655 (-474.699, -285.75) -> (-469.1998, -276.225)
  line L3656 (-455.4516, -255.5875) -> (-466.4501, -255.5875)
  line L3657 (-466.4501, -255.5875) -> (-471.9494, -265.1125)
  line L3658 (-471.9494, -265.1125) -> (-466.4501, -274.6375)
  line L3659 (-466.4501, -274.6375) -> (-455.4516, -274.6375)
  line L3660 (-449.9524, -265.1125) -> (-455.4516, -255.5875)
  line L3661 (-455.4516, -274.6375) -> (-449.9524, -265.1125)
  line L3662 (-436.2042, -244.475) -> (-447.2027, -244.475)
  line L3663 (-447.2027, -244.475) -> (-452.702, -254)
  line L3664 (-452.702, -254) -> (-447.2027, -263.525)
  line L3665 (-447.2027, -263.525) -> (-436.2042, -263.525)
  line L3666 (-430.7049, -254) -> (-436.2042, -244.475)
  line L3667 (-436.2042, -263.525) -> (-430.7049, -254)
  line L3668 (-416.9568, -233.3625) -> (-427.9553, -233.3625)
  line L3669 (-427.9553, -233.3625) -> (-433.4546, -242.8875)
  line L3670 (-433.4546, -242.8875) -> (-427.9553, -252.4125)
  line L3671 (-427.9553, -252.4125) -> (-416.9568, -252.4125)
  line L3672 (-411.4575, -242.8875) -> (-416.9568, -233.3625)
  line L3673 (-416.9568, -252.4125) -> (-411.4575, -242.8875)
  line L3674 (-397.7094, -222.25) -> (-408.7079, -222.25)
  line L3675 (-408.7079, -222.25) -> (-414.2072, -231.775)
  line L3676 (-414.2072, -231.775) -> (-408.7079, -241.3)
  line L3677 (-408.7079, -241.3) -> (-397.7094, -241.3)
  line L3678 (-392.2101, -231.775) -> (-397.7094, -222.25)
  line L3679 (-397.7094, -241.3) -> (-392.2101, -231.775)
  line L3680 (-378.462, -211.1375) -> (-389.4605, -211.1375)
  line L3681 (-389.4605, -211.1375) -> (-394.9597, -220.6625)
  line L3682 (-394.9597, -220.6625) -> (-389.4605, -230.1875)
  line L3683 (-389.4605, -230.1875) -> (-378.462, -230.1875)
  line L3684 (-372.9627, -220.6625) -> (-378.462, -211.1375)
  line L3685 (-378.462, -230.1875) -> (-372.9627, -220.6625)
  line L3686 (-359.2145, -200.025) -> (-370.2131, -200.025)
  line L3687 (-370.2131, -200.025) -> (-375.7123, -209.55)
  line L3688 (-375.7123, -209.55) -> (-370.2131, -219.075)
  line L3689 (-370.2131, -219.075) -> (-359.2145, -219.075)
  line L3690 (-353.7153, -209.55) -> (-359.2145, -200.025)
  line L3691 (-359.2145, -219.075) -> (-353.7153, -209.55)
  line L3692 (-339.9671, -188.9125) -> (-350.9657, -188.9125)
  line L3693 (-350.9657, -188.9125) -> (-356.4649, -198.4375)
  line L3694 (-356.4649, -198.4375) -> (-350.9657, -207.9625)
  line L3695 (-350.9657, -207.9625) -> (-339.9671, -207.9625)
  line L3696 (-334.4679, -198.4375) -> (-339.9671, -188.9125)
  line L3697 (-339.9671, -207.9625) -> (-334.4679, -198.4375)
  line L3698 (-320.7197, -177.8) -> (-331.7182, -177.8)
  line L3699 (-331.7182, -177.8) -> (-337.2175, -187.325)
  line L3700 (-337.2175, -187.325) -> (-331.7182, -196.85)
  line L3701 (-331.7182, -196.85) -> (-320.7197, -196.85)
  line L3702 (-315.2205, -187.325) -> (-320.7197, -177.8)
  line L3703 (-320.7197, -196.85) -> (-315.2205, -187.325)
  line L3704 (-301.4723, -166.6875) -> (-312.4708, -166.6875)
  line L3705 (-312.4708, -166.6875) -> (-317.9701, -176.2125)
  line L3706 (-317.9701, -176.2125) -> (-312.4708, -185.7375)
  line L3707 (-312.4708, -185.7375) -> (-301.4723, -185.7375)
  line L3708 (-295.973, -176.2125) -> (-301.4723, -166.6875)
  line L3709 (-301.4723, -185.7375) -> (-295.973, -176.2125)
  line L3710 (-282.2249, -155.575) -> (-293.2234, -155.575)
  line L3711 (-293.2234, -155.575) -> (-298.7227, -165.1)
  line L3712 (-298.7227, -165.1) -> (-293.2234, -174.625)
  line L3713 (-293.2234, -174.625) -> (-282.2249, -174.625)
  line L3714 (-276.7256, -165.1) -> (-282.2249, -155.575)
  line L3715 (-282.2249, -174.625) -> (-276.7256, -165.1)
  line L3716 (-262.9775, -144.4625) -> (-273.976, -144.4625)
  line L3717 (-273.976, -144.4625) -> (-279.4753, -153.9875)
  line L3718 (-279.4753, -153.9875) -> (-273.976, -163.5125)
  line L3719 (-273.976, -163.5125) -> (-262.9775, -163.5125)
  line L3720 (-257.4782, -153.9875) -> (-262.9775, -144.4625)
  line L3721 (-262.9775, -163.5125) -> (-257.4782, -153.9875)
  line L3722 (-243.7301, -133.35) -> (-254.7286, -133.35)
  line L3723 (-254.7286, -133.35) -> (-260.2278, -142.875)
  line L3724 (-260.2278, -142.875) -> (-254.7286, -152.4)
  line L3725 (-254.7286, -152.4) -> (-243.7301, -152.4)
  line L3726 (-238.2308, -142.875) -> (-243.7301, -133.35)
  line L3727 (-243.7301, -152.4) -> (-238.2308, -142.875)
  line L3728 (-224.4826, -122.2375) -> (-235.4812, -122.2375)
  line L3729 (-235.4812, -122.2375) -> (-240.9804, -131.7625)
  line L3730 (-240.9804, -131.7625) -> (-235.4812, -141.2875)
  line L3731 (-235.4812, -141.2875) -> (-224.4826, -141.2875)
  line L3732 (-218.9834, -131.7625) -> (-224.4826, -122.2375)
  line L3733 (-224.4826, -141.2875) -> (-218.9834, -131.7625)
  line L3734 (-205.2352, -111.125) -> (-216.2337, -111.125)
  line L3735 (-216.2337, -111.125) -> (-221.733, -120.65)
  line L3736 (-221.733, -120.65) -> (-216.2337, -130.175)
  line L3737 (-216.2337, -130.175) -> (-205.2352, -130.175)
  line L3738 (-199.736, -120.65) -> (-205.2352, -111.125)
  line L3739 (-205.2352, -130.175) -> (-199.736, -120.65)
  line L3740 (-185.9878, -100.0125) -> (-196.9863, -100.0125)
  line L3741 (-196.9863, -100.0125) -> (-202.4856, -109.5375)
  line L3742 (-202.4856, -109.5375) -> (-196.9863, -119.0625)
  line L3743 (-196.9863, -119.0625) -> (-185.9878, -119.0625)
  line L3744 (-180.4886, -109.5375) -> (-185.9878, -100.0125)
  line L3745 (-185.9878, -119.0625) -> (-180.4886, -109.5375)
  line L3746 (-166.7404, -88.9) -> (-177.7389, -88.9)
  line L3747 (-177.7389, -88.9) -> (-183.2382, -98.425)
  line L3748 (-183.2382, -98.425) -> (-177.7389, -107.95)
  line L3749 (-177.7389, -107.95) -> (-166.7404, -107.95)
  line L3750 (-161.2411, -98.425) -> (-166.7404, -88.9)
  line L3751 (-166.7404, -107.95) -> (-161.2411, -98.425)
  line L3752 (-147.493, -77.7875) -> (-158.4915, -77.7875)
  line L3753 (-158.4915, -77.7875) -> (-163.9908, -87.3125)
  line L3754 (-163.9908, -87.3125) -> (-158.4915, -96.8375)
  line L3755 (-158.4915, -96.8375) -> (-147.493, -96.8375)
  line L3756 (-141.9937, -87.3125) -> (-147.493, -77.7875)
  line L3757 (-147.493, -96.8375) -> (-141.9937, -87.3125)
  line L3758 (-128.2456, -66.675) -> (-139.2441, -66.675)
  line L3759 (-139.2441, -66.675) -> (-144.7434, -76.2)
  line L3760 (-144.7434, -76.2) -> (-139.2441, -85.725)
  line L3761 (-139.2441, -85.725) -> (-128.2456, -85.725)
  line L3762 (-122.7463, -76.2) -> (-128.2456, -66.675)
  line L3763 (-128.2456, -85.725) -> (-122.7463, -76.2)
  line L3764 (-108.9982, -55.5625) -> (-119.9967, -55.5625)
  line L3765 (-119.9967, -55.5625) -> (-125.4959, -65.0875)
  line L3766 (-125.4959, -65.0875) -> (-119.9967, -74.6125)
  line L3767 (-119.9967, -74.6125) -> (-108.9982, -74.6125)
  line L3768 (-103.4989, -65.0875) -> (-108.9982, -55.5625)
  line L3769 (-108.9982, -74.6125) -> (-103.4989, -65.0875)
  line L3770 (-89.7507, -44.45) -> (-100.7493, -44.45)
  line L3771 (-100.7493, -44.45) -> (-106.2485, -53.975)
  line L3772 (-106.2485, -53.975) -> (-100.7493, -63.5)
  line L3773 (-100.7493, -63.5) -> (-89.7507, -63.5)
  line L3774 (-84.2515, -53.975) -> (-89.7507, -44.45)
  line L3775 (-89.7507, -63.5) -> (-84.2515, -53.975)
  line L3776 (-70.5033, -33.3375) -> (-81.5018, -33.3375)
  line L3777 (-81.5018, -33.3375) -> (-87.0011, -42.8625)
  line L3778 (-87.0011, -42.8625) -> (-81.5018, -52.3875)
  line L3779 (-81.5018, -52.3875) -> (-70.5033, -52.3875)
  line L3780 (-65.0041, -42.8625) -> (-70.5033, -33.3375)
  line L3781 (-70.5033, -52.3875) -> (-65.0041, -42.8625)
  line L3782 (-51.2559, -22.225) -> (-62.2544, -22.225)
  line L3783 (-62.2544, -22.225) -> (-67.7537, -31.75)
  line L3784 (-67.7537, -31.75) -> (-62.2544, -41.275)
  line L3785 (-62.2544, -41.275) -> (-51.2559, -41.275)
  line L3786 (-45.7566, -31.75) -> (-51.2559, -22.225)
  line L3787 (-51.2559, -41.275) -> (-45.7566, -31.75)
  line L3788 (-32.0085, -11.1125) -> (-43.007, -11.1125)
  line L3789 (-43.007, -11.1125) -> (-48.5063, -20.6375)
  line L3790 (-48.5063, -20.6375) -> (-43.007, -30.1625)
  line L3791 (-43.007, -30.1625) -> (-32.0085, -30.1625)
  line L3792 (-26.5092, -20.6375) -> (-32.0085, -11.1125)
  line L3793 (-32.0085, -30.1625) -> (-26.5092, -20.6375)
  line L3794 (-12.7611, 0) -> (-23.7596, 0)
  line L3795 (-23.7596, 0) -> (-29.2589, -9.525)
  line L3796 (-29.2589, -9.525) -> (-23.7596, -19.05)
  line L3797 (-23.7596, -19.05) -> (-12.7611, -19.05)
  line L3798 (-7.2618, -9.525) -> (-12.7611, 0)
  line L3799 (-12.7611, -19.05) -> (-7.2618, -9.525)
  line L3800 (6.4863, 11.1125) -> (-4.5122, 11.1125)
  line L3801 (-4.5122, 11.1125) -> (-10.0114, 1.5875)
  line L3802 (-10.0114, 1.5875) -> (-4.5122, -7.9375)
  line L3803 (-4.5122, -7.9375) -> (6.4863, -7.9375)
  line L3804 (11.9856, 1.5875) -> (6.4863, 11.1125)
  line L3805 (6.4863, -7.9375) -> (11.9856, 1.5875)
  line L3806 (25.7337, 22.225) -> (14.7352, 22.225)
  line L3807 (14.7352, 22.225) -> (9.236, 12.7)
  line L3808 (9.236, 12.7) -> (14.7352, 3.175)
  line L3809 (14.7352, 3.175) -> (25.7337, 3.175)
  line L3810 (31.233, 12.7) -> (25.7337, 22.225)
  line L3811 (25.7337, 3.175) -> (31.233, 12.7)
  line L3812 (44.9812, 33.3375) -> (33.9826, 33.3375)
  line L3813 (33.9826, 33.3375) -> (28.4834, 23.8125)
  line L3814 (28.4834, 23.8125) -> (33.9826, 14.2875)
  line L3815 (33.9826, 14.2875) -> (44.9812, 14.2875)
  line L3816 (50.4804, 23.8125) -> (44.9812, 33.3375)
  line L3817 (44.9812, 14.2875) -> (50.4804, 23.8125)
  line L3818 (64.2286, 44.45) -> (53.2301, 44.45)
  line L3819 (53.2301, 44.45) -> (47.7308, 34.925)
  line L3820 (47.7308, 34.925) -> (53.2301, 25.4)
  line L3821 (53.2301, 25.4) -> (64.2286, 25.4)
  line L3822 (69.7278, 34.925) -> (64.2286, 44.45)
  line L3823 (64.2286, 25.4) -> (69.7278, 34.925)
  line L3824 (83.476, 55.5625) -> (72.4775, 55.5625)
  line L3825 (72.4775, 55.5625) -> (66.9782, 46.0375)
  line L3826 (66.9782, 46.0375) -> (72.4775, 36.5125)
  line L3827 (72.4775, 36.5125) -> (83.476, 36.5125)
  line L3828 (88.9753, 46.0375) -> (83.476, 55.5625)
  line L3829 (83.476, 36.5125) -> (88.9753, 46.0375)
  line L3830 (102.7234, 66.675) -> (91.7249, 66.675)
  line L3831 (91.7249, 66.675) -> (86.2256, 57.15)
  line L3832 (86.2256, 57.15) -> (91.7249, 47.625)
  line L3833 (91.7249, 47.625) -> (102.7234, 47.625)
  line L3834 (108.2227, 57.15) -> (102.7234, 66.675)
  line L3835 (102.7234, 47.625) -> (108.2227, 57.15)
  line L3836 (121.9708, 77.7875) -> (110.9723, 77.7875)
  line L3837 (110.9723, 77.7875) -> (105.473, 68.2625)
  line L3838 (105.473, 68.2625) -> (110.9723, 58.7375)
  line L3839 (110.9723, 58.7375) -> (121.9708, 58.7375)
  line L3840 (127.4701, 68.2625) -> (121.9708, 77.7875)
  line L3841 (121.9708, 58.7375) -> (127.4701, 68.2625)
  line L3842 (141.2182, 88.9) -> (130.2197, 88.9)
  line L3843 (130.2197, 88.9) -> (124.7205, 79.375)
  line L3844 (124.7205, 79.375) -> (130.2197, 69.85)
  line L3845 (130.2197, 69.85) -> (141.2182, 69.85)
  line L3846 (146.7175, 79.375) -> (141.2182, 88.9)
  line L3847 (141.2182, 69.85) -> (146.7175, 79.375)
  line L3848 (160.4657, 100.0125) -> (149.4671, 100.0125)
  line L3849 (149.4671, 100.0125) -> (143.9679, 90.4875)
  line L3850 (143.9679, 90.4875) -> (149.4671, 80.9625)
  line L3851 (149.4671, 80.9625) -> (160.4657, 80.9625)
  line L3852 (165.9649, 90.4875) -> (160.4657, 100.0125)
  line L3853 (160.4657, 80.9625) -> (165.9649, 90.4875)
  line L3854 (179.7131, 111.125) -> (168.7145, 111.125)
  line L3855 (168.7145, 111.125) -> (163.2153, 101.6)
  line L3856 (163.2153, 101.6) -> (168.7145, 92.075)
  line L3857 (168.7145, 92.075) -> (179.7131, 92.075)
  line L3858 (185.2123, 101.6) -> (179.7131, 111.125)
  line L3859 (179.7131, 92.075) -> (185.2123, 101.6)
  line L3860 (198.9605, 122.2375) -> (187.962, 122.2375)
  line L3861 (187.962, 122.2375) -> (182.4627, 112.7125)
  line L3862 (182.4627, 112.7125) -> (187.962, 103.1875)
  line L3863 (187.962, 103.1875) -> (198.9605, 103.1875)
  line L3864 (204.4597, 112.7125) -> (198.9605, 122.2375)
  line L3865 (198.9605, 103.1875) -> (204.4597, 112.7125)
  line L3866 (218.2079, 133.35) -> (207.2094, 133.35)
  line L3867 (207.2094, 133.35) -> (201.7101, 123.825)
  line L3868 (201.7101, 123.825) -> (207.2094, 114.3)
  line L3869 (207.2094, 114.3) -> (218.2079, 114.3)
  line L3870 (223.7072, 123.825) -> (218.2079, 133.35)
  line L3871 (218.2079, 114.3) -> (223.7072, 123.825)
  line L3872 (237.4553, 144.4625) -> (226.4568, 144.4625)
  line L3873 (226.4568, 144.4625) -> (220.9575, 134.9375)
  line L3874 (220.9575, 134.9375) -> (226.4568, 125.4125)
  line L3875 (226.4568, 125.4125) -> (237.4553, 125.4125)
  line L3876 (242.9546, 134.9375) -> (237.4553, 144.4625)
  line L3877 (237.4553, 125.4125) -> (242.9546, 134.9375)
  line L3878 (256.7027, 155.575) -> (245.7042, 155.575)
  line L3879 (245.7042, 155.575) -> (240.2049, 146.05)
  line L3880 (240.2049, 146.05) -> (245.7042, 136.525)
  line L3881 (245.7042, 136.525) -> (256.7027, 136.525)
  line L3882 (262.202, 146.05) -> (256.7027, 155.575)
  line L3883 (256.7027, 136.525) -> (262.202, 146.05)
  line L3884 (275.9501, 166.6875) -> (264.9516, 166.6875)
  line L3885 (264.9516, 166.6875) -> (259.4524, 157.1625)
  line L3886 (259.4524, 157.1625) -> (264.9516, 147.6375)
  line L3887 (264.9516, 147.6375) -> (275.9501, 147.6375)
  line L3888 (281.4494, 157.1625) -> (275.9501, 166.6875)